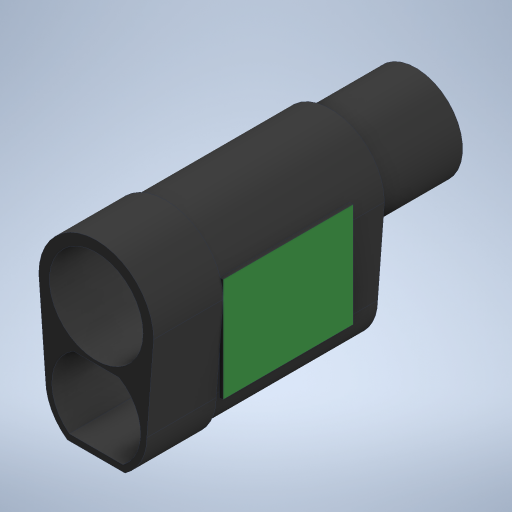
# Autodesk Inventor part: Big LRF Real
Saved by Autodesk Inventor 2024.1 (Build 281209000, 209)
## iProperties
Created: 2025-04-08
Part Number: Big LRF Real
Material: Generic
Document SubType Name: Modeling
Designer: User
Density: 1 g/cm^3
Appearance: Rubber - Blue
Author: User
Autodesk Inventor part; units mm, degrees
ref_plane "YZ Plane" through (0, 0, 0) normal (1, 0, 0) x (0, 1, 0)
ref_plane "XZ Plane" through (0, 0, 0) normal (0, 1, 0) x (-1, 0, 0)
ref_plane "XY Plane" through (0, 0, 0) normal (0, 0, 1) x (1, 0, 0)
sketch "Sketch1" plane through (0, 0, 0) normal (0, 0, 1) x (1, 0, 0)
  line L0 (0, 0) -> (33.1, 0)
  line L1 (33.1, 0) -> (33.1, 54)
  line L2 (33.1, 54) -> (0, 54)
  line L3 (0, 54) -> (0, 0)
  arc A0 (32.9068, 34.9287) -> (0.1932, 34.9287) centre (16.55, 37.45) ccw
  line L4 (0, 37.45) -> (1.95, 12)
  line L5 (1.95, 12) -> (13.9851, 12) construction
  line L6 (8.2338, 0) -> (24.8662, 0)
  line L7 (33.1, 37.45) -> (31.15, 12)
  arc A1 (1.95, 12) -> (8.2338, 0) centre (16.55, 12) ccw
  arc A2 (24.8662, 0) -> (31.15, 12) centre (16.55, 12) ccw
  dimension "d0" = 33.1
  dimension "d1" = 54
  dimension "d2" = 33.1
  constraints: 16 end point, 8 point on circle, 6 point on line, 3 centre point, 2 horizontal, 2 parallel, 1 perpendicular
  measures "d0" distance of L2.end L1.end
  measures "d1" distance of L1.end L0.end
  measures "d2" diameter of A0
extrude "Extrusion1" add sketch "Sketch1" against normal blind 67.52 contours A1 L4 A0 L7 A2 L0
sketch "Sketch3" plane through (0, 0, 0) normal (0, 0, 1) x (1, 0, 0)
  arc A0 (33.1, 37.45) -> (0, 37.45) centre (16.55, 37.45) ccw projected
  circle A1 centre (16.55, 37.45) radius 13.5
  arc A2 (24.8662, 0) -> (31.15, 12) centre (16.55, 12) ccw projected
  line L0 (8.817, 1.8) -> (24.283, 1.8)
  line L1 (8.817, 1.8) -> (24.283, 1.8) construction
  line L2 (10.0048, 23) -> (23.0952, 23)
  arc A3 (10.0048, 23) -> (8.817, 1.8) centre (16.55, 12) ccw
  arc A4 (24.283, 1.8) -> (23.0952, 23) centre (16.55, 12) ccw
  point P0 (0, 0)
  dimension "d7" = 27
  constraints: 6 end point, 5 point on circle, 3 centre point, 2 coincident, 2 horizontal, 1 collinear
  measures "d7" diameter of A1
extrude "Extrusion2" cut sketch "Sketch3" against normal blind 56.52
sketch "Sketch4" plane through (0, 0, -67.52) normal (0, 0, -1) x (-1, 0, 0)
  arc A0 (0, 37.45) -> (-33.1, 37.45) centre (-16.55, 37.45) ccw projected
  circle A1 centre (-16.55, 37.45) radius 13.5
  point P0 (0, 0)
  constraints: 1 centre point, 1 coincident
extrude "Extrusion3" add sketch "Sketch4" along normal blind 24.59
sketch "Sketch7" plane through (0, 0, -67.52) normal (0, 0, -1) x (-1, 0, 0)
  circle A0 centre (-16.55, 37.45) radius 13.5 projected
  arc A1 (0, 37.45) -> (-33.1, 37.45) centre (-16.55, 37.45) ccw
  arc A2 (-23.0952, 23) -> (-24.283, 1.8) centre (-16.55, 12) ccw projected
  line L0 (-1.95, 12) -> (0, 37.45)
  line L1 (-24.8662, 0) -> (-8.2338, 0) projected
  line L2 (-24.8662, 0) -> (-8.2338, 0)
  arc A3 (-8.2338, 0) -> (-1.95, 12) centre (-16.55, 12) ccw
  arc A4 (-31.15, 12) -> (-24.8662, 0) centre (-16.55, 12) ccw
  arc A5 (-31.15, 12) -> (-24.8662, 0) centre (-16.55, 12) ccw projected
  line L3 (-31.15, 12) -> (-33.1, 37.45)
  arc A6 (-1, 37.4877) -> (-32.1, 37.45) centre (-16.55, 37.45) ccw
  line L4 (-1, 37.4877) -> (-2.9501, 12.0376)
  arc A7 (-8.5525, 1) -> (-2.9501, 12.0376) centre (-16.55, 12) ccw
  line L5 (-8.5525, 1) -> (-24.5475, 1)
  arc A8 (-30.1499, 12.0376) -> (-24.5475, 1) centre (-16.55, 12) ccw
  line L6 (-30.1499, 12.0376) -> (-32.1029, 37.5264)
  point P0 (0, 0)
  point P1 (-32.1, 37.4877)
  dimension "d21" = 1
  constraints: 12 end point, 12 point on circle, 6 centre point, 2 coincident, 1 collinear, 1 point on line, 5 other
  measures "d21" radial gap between concentric circles of A1 A6
extrude "Extrusion6" cut sketch "Sketch7" against normal blind 47.52 contours L0 A3 L1 A4 L3 A1
sketch "Sketch8" plane through (16.55, 37.45, -92.11) normal (0, 0, -1) x (-1, 0, 0)
  circle A0 centre (0, 0) radius 11.5
  point P0 (16.55, -37.45)
  dimension "d24" = 23
  constraints: 1 centre point
  measures "d24" diameter of A0
extrude "Extrusion7" cut sketch "Sketch8" against normal blind 44.77
sketch "Sketch11" plane through (0, 0, -67.52) normal (0, 0, -1) x (-1, 0, 0)
  arc A0 (0, 37.45) -> (-33.1, 37.45) centre (-16.55, 37.45) ccw projected
  line L0 (-33.1, 37.45) -> (-28.1, 37.45) construction
  line L1 (-33.1, 12.45) -> (-32.1, 12.45)
  line L2 (-32.1, 12.45) -> (-32.1, 42.45)
  line L3 (-32.1, 42.45) -> (-33.1, 42.45)
  line L4 (-33.1, 42.45) -> (-33.1, 12.45)
  point P0 (0, 0)
  dimension "d39" = 1
  constraints: 10 end point, 2 horizontal, 2 parallel, 1 perpendicular
  measures "d39" distance of L3.end L2.end
extrude "Extrusion9" add sketch "Sketch11" against normal blind 47.52
sketch "Sketch12" plane through (0, 0, -67.52) normal (0, 0, -1) x (-1, 0, 0)
  line L0 (-32.1, 12.45) -> (-33.1, 12.45) projected
  line L1 (-32.1, 42.45) -> (-32.1, 24.3987) projected
  line L2 (-33.1, 12.45) -> (-32.1, 12.45)
  line L3 (-32.1, 12.45) -> (-32.1, 42.45)
  line L4 (-32.1, 42.45) -> (-33.1, 42.45)
  line L5 (-33.1, 42.45) -> (-33.1, 12.45)
  point P0 (0, 0)
  constraints: 8 end point, 2 parallel, 1 horizontal, 1 perpendicular
extrude "Extrusion10" cut sketch "Sketch12" against normal blind 10
body "Solid1"
